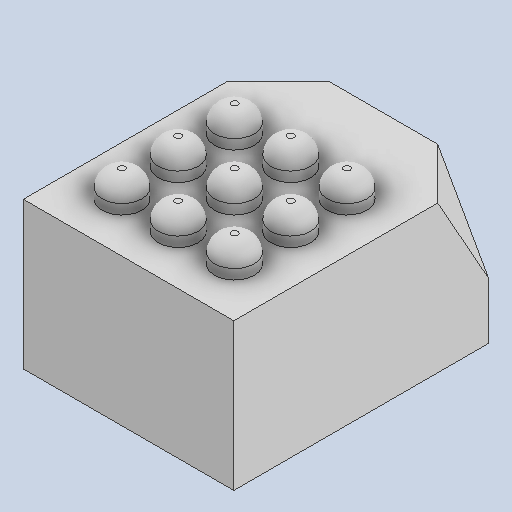
# Autodesk Inventor part: Contactile Sensor
Saved by Autodesk Inventor 2022 (Build 260153000, 153)
## iProperties
Created: 2021-09-24
Part Number: Contactile Sensor
Material: Generic
Document SubType Name: Modeling
Designer: kylem
Density: 1 g/cm^3
Appearance: Default
Author: kylem
Autodesk Inventor part; units mm, degrees
ref_plane "YZ Plane" through (0, 0, 0) normal (1, 0, 0) x (0, 1, 0)
sketch "Sketch1" plane through (0, 0, 0) normal (0, 1, 0) x (-1, 0, 0)
  line L0 (0, 0) -> (31.8, 0)
  line L1 (31.8, 0) -> (31.8, -38.5)
  line L2 (31.8, -38.5) -> (0, -38.5)
  line L3 (0, -38.5) -> (0, 0)
  dimension "d0" = 31.8
  dimension "d1" = 38.5
  constraints: 8 end point, 2 parallel, 1 horizontal, 1 perpendicular
  measures "d0" distance of L1.end L2.end
  measures "d1" distance of L0.end L1.end
extrude "Extrusion1" add sketch "Sketch1" along normal blind 22.2
sketch "Sketch2" plane through (0, 0, 0) normal (0, -1, 0) x (1, 0, 0)
  line L0 (-31.8, 0) -> (0, 0) projected
  line L1 (-15.9, 0) -> (-15.9, -1.476)
  line L2 (-15.9, 0) -> (-15.9, -16)
  line L3 (-15.9, -16) -> (-5.9, -16)
  line L4 (-5.9, -16) -> (-25.9, -16)
  line L5 (-15.9, -16) -> (-15.9, -26)
  line L6 (-15.9, -26) -> (-15.9, -6)
  circle A0 centre (-15.9, -6) radius 1.5
  circle A1 centre (-5.9, -16) radius 1.5
  circle A2 centre (-15.9, -26) radius 1.5
  circle A3 centre (-25.9, -16) radius 1.5
  dimension "d4" = 16
  dimension "d5" = 10
  dimension "d6" = 20
  dimension "d7" = 10
  dimension "d8" = 20
  dimension "d9" = 3
  dimension "d10" = 3
  dimension "d11" = 3
  dimension "d12" = 3
  constraints: 12 end point, 4 centre point, 4 coincident, 3 vertical, 2 point on line, 1 midpoint, 1 perpendicular
  measures "d4" distance of L1.start L2.end
  measures "d5" distance of L2.end L3.end
  measures "d6" distance of L3.end L4.end
  measures "d7" distance of L2.end L5.end
  measures "d8" distance of L5.end L6.end
  measures "d9" diameter of A0
  measures "d10" diameter of A1
  measures "d11" diameter of A2
  measures "d12" diameter of A3
extrude "Extrusion2" cut sketch "Sketch2" against normal blind 4.5
sketch "Sketch3" plane through (0, 22.2, 0) normal (0, 1, 0) x (1, 0, 0)
  line L0 (-31.8, 0) -> (0, 0) projected
  line L1 (-15.9, 0) -> (-15.9, 16)
  circle A0 centre (-15.9, 16) radius 3
  circle A1 centre (-7.4, 16) radius 3
  circle A2 centre (-24.4, 16) radius 3
  circle A3 centre (-7.4, 7.5) radius 3
  circle A4 centre (-15.9, 7.5) radius 3
  circle A5 centre (-24.4, 7.5) radius 3
  circle A6 centre (-7.4, 24.5) radius 3
  circle A7 centre (-15.9, 24.5) radius 3
  circle A8 centre (-24.4, 24.5) radius 3
  dimension "d15" = 16
  dimension "d16" = 6
  dimension "d19" = 8.5
  dimension "d26" = 8.5
  dimension "d33" = 8.5
  dimension "d40" = 8.5
  constraints: 9 centre point, 3 vertical, 2 end point, 2 horizontal, 1 coincident, 1 midpoint, 16 other
  measures "d15" distance of L1.start L1.end
  measures "d16" diameter of A0
  measures "d19" distance of A0.centre A1.centre
  measures "d26" distance of A0.centre A2.centre
  measures "d33" distance of A1.centre A3.centre
  measures "d40" distance of A1.centre A6.centre
extrude "Extrusion3" add sketch "Sketch3" along normal blind 4
fillet "Fillet1" radius 2.5 9 edges at (-10.4, 26.2, -7.5) (-18.9, 26.2, -7.5) (-27.4, 26.2, -7.5) (-27.4, 26.2, -16) (-18.9, 26.2, -16) (-10.4, 26.2, -16) (-10.4, 26.2, -24.5) (-18.9, 26.2, -24.5) (-27.4, 26.2, -24.5)
sketch "Sketch4" plane through (0, 0, -38.5) normal (0, 0, -1) x (-1, 0, 0)
  line L0 (17.4, 0) -> (14.4, 0) projected
  line L1 (15.9, 0) -> (15.9, 12)
  line L2 (15.9, 12) -> (24.3, 12)
  line L3 (15.9, 12) -> (24.3, 12) construction
  line L4 (24.3, 12) -> (7.5, 12)
  line L5 (7.5, 12) -> (7.5, 8.2)
  line L6 (7.5, 8.2) -> (24.3, 8.2)
  line L7 (24.3, 8.2) -> (24.3, 12)
  point P0 (0, 0)
  dimension "d48" = 12
  dimension "d49" = 8.4
  dimension "d50" = 0
  dimension "d51" = 16.8
  dimension "d52" = 3.8
  constraints: 14 end point, 3 horizontal, 2 parallel, 1 collinear, 1 midpoint, 1 perpendicular, 1 vertical
  measures "d48" distance of L1.start L1.end
  measures "d49" distance of L1.end L2.end
  measures "d50" distance between parallel lines of L2 L3
  measures "d51" distance of L6.end L5.end
  measures "d52" distance of L5.end L4.end
extrude "Extrusion4" cut sketch "Sketch4" against normal blind 6
sketch3d "3D Sketch1"
ref_plane "Work Plane1" through (0, 22.2, -30.8) normal (-0.6571, -0.3693, 0.6571) x (-0.7071, 0, -0.7071)
sketch "Sketch5" plane through (0, 22.2, -30.8) normal (-0.6571, -0.3693, 0.6571) x (-0.7071, 0, -0.7071)
  line L0 (-21.7789, -8.0435) -> (5.4447, 2.0109) projected
  line L1 (-3.5227, -1.301) -> (16.1237, -1.301)
  line L2 (16.1237, -1.301) -> (16.1237, 19.91)
  line L3 (16.1237, 19.91) -> (-3.5227, 19.91)
  line L4 (-3.5227, 19.91) -> (-3.5227, -1.301)
  point P0 (-21.7789, 12.5869)
  constraints: 8 end point, 2 parallel, 1 horizontal, 1 perpendicular, 1 point on line
extrude "Extrusion5" cut sketch "Sketch5" against normal blind 6
ref_plane "Work Plane2" through (-15.9, 0, -38.5) normal (-1, 0, 0) x (0, 0, 1)
mirror "Mirror1" about plane through (-15.9, 0, -38.5) normal (-1, 0, 0) of "Extrusion5"
body "Solid1"
